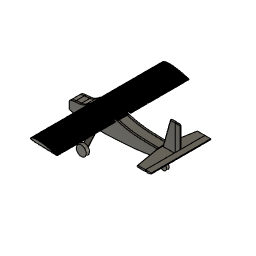
Arduino RC Plane - 3D Model (Autodesk Fusion 360 design; units mm, degrees)
Autodesk Fusion 360 part; units mm, degrees
(part 1 of 2)
sketch "Sketch1" plane through (0, 0, 0) normal (0, 1, 0) x (1, 0, 0)
  line L0 (95.8934, 1.764) -> (92.7195, 0.9111)
  line L1 (8.2584, 6.4801) -> (11.4851, 6.5775)
  line L2 (16.0241, -12.0922) -> (12.8008, -12.2387)
  line L3 (35.3144, -10.5067) -> (32.1062, -10.869)
  line L4 (14.7111, 6.6848) -> (17.9371, 6.7921)
  line L5 (12.8008, -12.2387) -> (9.5755, -12.3558)
  line L6 (37.2933, 7.4358) -> (40.5193, 7.5431)
  line L7 (34.0673, 7.3285) -> (37.2933, 7.4358)
  line L8 (27.6152, 7.114) -> (30.8412, 7.2213)
  line L9 (21.1632, 6.8994) -> (24.3892, 7.0067)
  line L10 (80.0088, -2.2846) -> (76.8274, -3.0295)
  line L11 (72.7795, 8.616) -> (76.0056, 8.7233)
  line L12 (40.5193, 7.5431) -> (43.7453, 7.6504)
  line L13 (38.5205, -10.1149) -> (35.3144, -10.5067)
  line L14 (88.9103, 9.1426) -> (92.1364, 9.2499)
  line L15 (24.3892, 7.0067) -> (27.6152, 7.114)
  line L16 (51.321, -8.2044) -> (48.1238, -8.7237)
  line L17 (-27.9436, -7.5856) -> (-29.6101, -6.8741)
  line L18 (44.9246, -9.2136) -> (41.7239, -9.6838)
  line L19 (92.1364, 9.2499) -> (95.3624, 9.3572)
  line L20 (53.4234, 7.9723) -> (56.6494, 8.0795)
  line L21 (-6.6136, -12.0485) -> (-9.8712, -11.7045)
  line L22 (-22.9804, -9.2004) -> (-26.284, -8.1991)
  line L23 (60.9003, -6.4698) -> (57.7093, -7.0774)
  line L24 (-11.0841, 5.6401) -> (-7.8642, 5.8357)
  line L25 (-30.3263, 3.3679) -> (-28.7346, 3.7257)
  line L26 (111.4925, 9.8936) -> (114.7185, 10.0009)
  line L27 (-23.9353, 4.4556) -> (-20.7278, 4.8278)
  line L28 (-3.3643, -12.2748) -> (-6.6136, -12.0485)
  line L29 (-33.4961, 2.4562) -> (-31.914, 2.9513)
  line L30 (59.8754, 8.1868) -> (63.1015, 8.2941)
  line L31 (56.6494, 8.0795) -> (59.8754, 8.1868)
  line L32 (-35.9566, 0.7068) -> (-35.3615, 1.3596)
  line L33 (118.0804, 8.1657) -> (114.9147, 7.1951)
  line L34 (-9.8712, -11.7045) -> (-13.1356, -11.2624)
  line L35 (9.5755, -12.3558) -> (6.3474, -12.4336)
  line L36 (30.8412, 7.2213) -> (34.0673, 7.3285)
  line L37 (108.5786, 5.3226) -> (105.4096, 4.4011)
  line L38 (48.1238, -8.7237) -> (44.9246, -9.2136)
  line L39 (50.1974, 7.865) -> (53.4234, 7.9723)
  line L40 (79.2323, 8.8207) -> (82.4583, 8.928)
  line L41 (63.1015, 8.2941) -> (66.3275, 8.4014)
  line L42 (22.4652, -11.7206) -> (19.246, -11.926)
  line L43 (122.7836, 10.2691) -> (125.1135, 10.3466)
  line L44 (-35.7385, -2.4129) -> (-36.0972, -1.9352)
  line L45 (-36.4605, -0.265) -> (-36.3957, -0.0633)
  line L46 (-17.5162, 5.1411) -> (-14.3018, 5.4151)
  line L47 (-35.0466, -3.1433) -> (-35.7385, -2.4129)
  line L48 (85.6843, 9.0353) -> (88.9103, 9.1426)
  line L49 (69.5535, 8.5087) -> (72.7795, 8.616)
  line L50 (5.0323, 6.3728) -> (8.2584, 6.4801)
  line L51 (122.8282, 9.6314) -> (121.2454, 9.1461)
  line L52 (28.8953, -11.1921) -> (25.6816, -11.476)
  line L53 (-36.0972, -1.9352) -> (-36.2873, -1.6133)
  line L54 (-7.8642, 5.8357) -> (-4.6423, 6.0019)
  line L55 (6.3474, -12.4336) -> (3.1152, -12.4526)
  line L56 (-27.138, 4.0148) -> (-23.9353, 4.4556)
  line L57 (98.5884, 9.4645) -> (101.8144, 9.5717)
  line L58 (57.7093, -7.0774) -> (54.5162, -7.6556)
  line L59 (125.1135, 10.3466) -> (122.8282, 9.6314)
  line L60 (-29.6101, -6.8741) -> (-31.2876, -6.0056)
  line L61 (119.5576, 10.1618) -> (121.1706, 10.2155)
  line L62 (64.0893, -5.8328) -> (60.9003, -6.4698)
  line L63 (92.7195, 0.9111) -> (89.5435, 0.0876)
  line L64 (-13.1356, -11.2624) -> (-16.4076, -10.7124)
  line L65 (111.747, 6.254) -> (108.5786, 5.3226)
  line L66 (119.6632, 8.651) -> (118.0804, 8.1657)
  line L67 (89.5435, 0.0876) -> (86.3669, -0.726)
  line L68 (121.1706, 10.2155) -> (122.7836, 10.2691)
  line L69 (-36.3957, -0.0633) -> (-36.2502, 0.2525)
  line L70 (-34.7442, 1.8366) -> (-33.4961, 2.4562)
  line L71 (76.0056, 8.7233) -> (79.2323, 8.8207)
  line L72 (114.9147, 7.1951) -> (111.747, 6.254)
  line L73 (-36.2873, -1.6133) -> (-36.3816, -1.3932)
  line L74 (95.3624, 9.3572) -> (98.5884, 9.4645)
  line L75 (67.2762, -5.1663) -> (64.0893, -5.8328)
  line L76 (102.2384, 3.5089) -> (99.0666, 2.6266)
  line L77 (-35.3615, 1.3596) -> (-34.7442, 1.8366)
  line L78 (-20.7278, 4.8278) -> (-17.5162, 5.1411)
  line L79 (114.7185, 10.0009) -> (117.9446, 10.1082)
  line L80 (-14.3018, 5.4151) -> (-11.0841, 5.6401)
  line L81 (-36.4861, -1.0259) -> (-36.4605, -0.265)
  line L82 (-31.2876, -6.0056) -> (-32.983, -4.882)
  line L83 (-34.3525, -3.7651) -> (-35.0466, -3.1433)
  line L84 (117.9446, 10.1082) -> (119.5576, 10.1618)
  line L85 (-32.983, -4.882) -> (-34.3525, -3.7651)
  line L86 (105.0405, 9.679) -> (108.2665, 9.7863)
  line L87 (-26.284, -8.1991) -> (-27.9436, -7.5856)
  line L88 (70.4618, -4.4802) -> (67.2762, -5.1663)
  line L89 (66.3275, 8.4014) -> (69.5535, 8.5087)
  line L90 (-28.7346, 3.7257) -> (-27.138, 4.0148)
  line L91 (-16.4076, -10.7124) -> (-19.6885, -10.0349)
  line L92 (108.2665, 9.7863) -> (111.4925, 9.8936)
  line L93 (43.7453, 7.6504) -> (46.9713, 7.7577)
  line L94 (76.8274, -3.0295) -> (73.6453, -3.7647)
  line L95 (54.5162, -7.6556) -> (51.321, -8.2044)
  line L96 (-36.3816, -1.3932) -> (-36.4861, -1.0259)
  line L97 (101.8144, 9.5717) -> (105.0405, 9.679)
  line L98 (105.4096, 4.4011) -> (102.2384, 3.5089)
  line L99 (46.9713, 7.7577) -> (50.1974, 7.865)
  line L100 (73.6453, -3.7647) -> (70.4618, -4.4802)
  line L101 (-36.2502, 0.2525) -> (-35.9566, 0.7068)
  line L102 (-31.914, 2.9513) -> (-30.3263, 3.3679)
  line L103 (99.0666, 2.6266) -> (95.8934, 1.764)
  line L104 (-1.4183, 6.1386) -> (1.8063, 6.2655)
  line L105 (83.1882, -1.5102) -> (80.0088, -2.2846)
  line L106 (86.3669, -0.726) -> (83.1882, -1.5102)
  line L107 (19.246, -11.926) -> (16.0241, -12.0922)
  line L108 (121.2454, 9.1461) -> (119.6632, 8.651)
  line L109 (-4.6423, 6.0019) -> (-1.4183, 6.1386)
  line L110 (25.6816, -11.476) -> (22.4652, -11.7206)
  line L111 (1.8063, 6.2655) -> (5.0323, 6.3728)
  line L112 (17.9371, 6.7921) -> (21.1632, 6.8994)
  line L113 (-19.6885, -10.0349) -> (-22.9804, -9.2004)
  line L114 (41.7239, -9.6838) -> (38.5205, -10.1149)
  line L115 (11.4851, 6.5775) -> (14.7111, 6.6848)
  line L116 (3.1152, -12.4526) -> (-0.1211, -12.4128)
  line L117 (82.4583, 8.928) -> (85.6843, 9.0353)
  line L118 (-0.1211, -12.4128) -> (-3.3643, -12.2748)
  line L119 (32.1062, -10.869) -> (28.8953, -11.1921)
  line L120 (433.5139, 105.8779) -> (-166.4861, 105.8779) construction
  line L121 (369.1135, 36.3466) -> (475.1135, 36.3466)
  line L122 (475.1135, 36.3466) -> (475.1135, 46.3466)
  line L123 (475.1135, 46.3466) -> (369.1135, 46.3466)
  line L124 (365.1135, 42.3466) -> (365.1135, 40.3466)
  arc A0 (365.1135, 40.3466) -> (369.1135, 36.3466) centre (369.1135, 40.3466) ccw
  arc A1 (369.1135, 46.3466) -> (365.1135, 42.3466) centre (369.1135, 42.3466) ccw
  line L125 (433.5395, 58.3466) -> (433.5395, 46.3466)
  line L126 (-36.4605, -0.265) -> (-72.4401, 24.9282)
  line L127 (-36.4605, -0.265) -> (0.5767, -0.265) construction
  line L128 (-101.6254, 35.5508) -> (-134.5473, 38.4311)
  line L129 (-166.4605, 53.4227) -> (-166.4605, 88.4227)
  spline S0 degree 5 poles (-158.5986, 98.1914) (-149.6531, 100.1493) (-132.0524, 103.7409) (-106.5214, 108.1556) (-73.5167, 112.2028) (-30.3842, 114.7027) (18.5122, 115.149) (75.7604, 113.8377) (140.9642, 110.664) (211.8798, 105.2223) (285.3301, 96.9119) (343.4794, 87.4326) (385.5551, 78.4692) (412.7641, 71.6318) (426.1581, 67.9976) knots 0 0 0 0 0 0 0.1 0.2 0.3 0.4 0.5 0.6 0.7 0.8 0.9 1 1 1 1 1 1
  line L130 (-201.7693, -33.0131) -> (-201.7693, 169.9869) construction
  line L131 (-201.7693, 68.4869) -> (-175.4519, 68.4869) construction
  arc A2 (-72.4401, 24.9282) -> (-101.6254, 35.5508) centre (-106.8547, -24.2209) ccw
  arc A3 (-159.8637, 44.0196) -> (-134.5473, 38.4311) centre (-125.8317, 138.0506) ccw
  arc A4 (-166.4605, 53.4227) -> (-159.8637, 44.0196) centre (-156.4605, 53.4227) ccw
  arc A5 (-158.5986, 98.1914) -> (-166.4605, 88.4227) centre (-156.4605, 88.4227) ccw
  arc A6 (433.5395, 58.3466) -> (426.1581, 67.9976) centre (423.5395, 58.3466) ccw
  line L132 (108.2665, 9.7863) -> (108.2665, 5.2318)
  spline S1 degree 5 poles (125.1135, 10.3466) (129.5122, 11.7241) (138.3251, 14.3811) (151.5908, 18.0725) (169.3737, 22.3977) (191.7903, 26.7637) (214.4829, 30.0801) (237.5863, 32.3933) (261.3798, 33.9707) (286.0084, 35.049) (311.4928, 35.7657) (332.5461, 36.1182) (348.6931, 36.2739) (359.614, 36.3302) (365.1135, 36.3466) knots 0 0 0 0 0 0 0.1 0.2 0.3 0.4 0.5 0.6 0.7 0.8 0.9 1 1 1 1 1 1
  line L133 (209.1359, 29.5835) -> (254.6924, 33.8044)
  line L134 (365.1135, 36.3466) -> (365.1135, 46.3466)
  spline S2 degree 5 poles (365.1135, 46.3466) (365.2736, 46.3477) (365.5937, 46.3495) (366.0739, 46.3513) (366.7139, 46.3521) (367.5139, 46.3513) (368.1538, 46.3498) (368.6336, 46.3483) (368.9536, 46.3472) (369.1135, 46.3466) knots 0 0 0 0 0 0 0.2 0.4 0.6 0.8 1 1 1 1 1 1
  line L135 (364.7053, 46.3438) -> (365.5217, 46.3493)
  line L136 (369.1135, 36.3466) -> (413.4661, -123.6534)
  line L137 (413.4661, -123.6534) -> (475.1135, -123.6534)
  line L138 (475.1135, -123.6534) -> (475.1135, 36.3466)
  point P0 (365.1135, 36.3466)
  point P1 (365.1135, 46.3466)
  point P2 (-85.6096, 34.1496)
  point P3 (-146.7743, 39.5008)
  point P4 (-166.4605, 100.9441)
  point P5 (19.9322, 114.7113)
  point P6 (433.5395, 70.3466)
  point P7 (231.9141, 31.694)
  dimension "d2" = 600
  dimension "d3" = 130
  dimension "d4" = 110
  dimension "d5" = 10
  dimension "d6" = 240
  dimension "d7" = 4
  dimension "d8" = 26
  dimension "d9" = 145
  dimension "d10" = 60
  dimension "d11" = 150
  dimension "d15" = 130
  dimension "d18" = 203
  dimension "d20" = 60
  dimension "d21" = 100
  dimension "d22" = 10
  dimension "d23" = 10
  dimension "d24" = 600
  dimension "d25" = 10
  dimension "d26" = 35
  dimension "d60" = 12
  dimension "d61" = 160
  constraint horizontal L120
  constraint horizontal L121
  constraint vertical L122
  constraint horizontal L123
  constraint vertical L124
  constraint coincident P0 L124
  constraint coincident P0 L121
  constraint tangent L124 A0
  constraint tangent L121 A0
  constraint coincident P1 L123
  constraint coincident P1 L124
  constraint tangent L123 A1
  constraint tangent L124 A1
  constraint equal A0 A1
  constraint coincident L123 L125.end
  constraint perpendicular L123 L125
  constraint horizontal L127
  constraint vertical L129
  constraint vertical L130
  constraint midpoint L130 L131.start
  constraint perpendicular L130 L131
  constraint coincident P2 L128
  constraint coincident P2 L126
  constraint tangent L128 A2
  constraint tangent L126 A2
  constraint coincident P3 L128
  constraint tangent L128 A3
  constraint tangent L129 A4
  constraint tangent A3 A4
  constraint coincident P4 L129
  constraint tangent L129 A5
  constraint tangent S0 A5
  constraint coincident L125 P6
  constraint tangent S0 A6
  constraint tangent L125 A6
  constraint vertical L132
  constraint coincident L37 L132.end
  constraint coincident P0 S1.end
  constraint midpoint P7 L133
  constraint coincident P1 L134.end
  constraint coincident L134 P1
  constraint midpoint P1 L135
  constraint perpendicular L125 L137
  constraint perpendicular L121 L138
  measures "d2" distance of L120.start L120.end
  measures "d3" horizontal distance of L81.start L120.end
  measures "d4" distance of P0 L121.end
  measures "d5" distance of P0 P1
  measures "d6" distance of L43.end L124
  measures "d7" radius of A0
  measures "d8" distance of L43.end L121
  measures "d9" angle of L126 L127
  measures "d10" distance of L45.start P2
  measures "d11" angle of L126 L128
  measures "d15" distance of L45.start L129
  measures "d18" distance of L130.start L130.end
  measures "d20" radius of A2
  measures "d21" radius of A3
  measures "d22" radius of A4
  measures "d23" radius of A5
  measures "d24" distance of L125 L129
  measures "d25" radius of A6
  measures "d26" distance of L129.start L129.end
  measures "d60" distance of L125.end L125.start
  measures "d61" distance of L121.end L137.end
extrude "Extrude1" add sketch "Sketch1" along normal mid plane 800 contours L0 L1 L2 L3 L4 L5 L6 L7 L8 L9 L10 L11 L12 L13 L14 L15 L16 L17 L18 L19 L20 L21 L22 L23 L24 L25 L27 L28 L29 L30 L31 L32 L34 L35 L36 L37 L38 L39 L40 L41 L42 L44 L45 L46 L47 L48 L49 L50 L52 L53 L54 L55 L56 L57 L58 L60 L62 L63 L64 L67 L69 L70 L71 L73 L74 L75 L76 L77 L78 L80 L81 L82 L83 L85 L86 L87 L88 L89 L90 L91 L93 L94 L95 L96 L97 L98 L99 L100 L101 L102 L103 L104 L105 L106 L107 L109 L110 L111 L112 L113 L114 L115 L116 L117 L118 L119 L132 | L26 L33 L37 L43 L51 L59 L61 L65 L66 L68 L72 L79 L84 L92 L108 L132 makes body 1
copy_body "Body->Comp2" bodies 1 removing the originals makes body 2 in component "Component"
extrude "Extrude1'" add sketch "Sketch1" along normal blind 45 separate body contours L1 L4 L6 L7 L8 L9 L11 L12 L14 L15 L19 L20 L24 L25 L26 L27 L29 L30 L31 L32 L36 L39 L40 L41 L43 L45 L46 L48 L49 L50 L54 L56 L57 L61 L68 L69 L70 L71 L74 L77 L78 L79 L80 L84 L86 L89 L90 L92 L93 L97 L99 L101 L102 L104 L109 L111 L112 L115 L117 L123 L124 L125 L126 L128 L129 S0 A2 A3 A4 A5 A6 S1 L134 S2 L135 makes body 3 in component "Component'"
extrude "Extrude2" cut sketch "Sketch1" along normal blind 25 contours L1 L4 L6 L7 L8 L9 L11 L12 L14 L15 L19 L20 L24 L25 L26 L27 L29 L30 L31 L32 L36 L39 L40 L41 L43 L45 L46 L48 L49 L50 L54 L56 L57 L61 L68 L69 L70 L71 L74 L77 L78 L79 L80 L84 L86 L89 L90 L92 L93 L97 L99 L101 L102 L104 L109 L111 L112 L115 L117 L123 L124 L125 L126 L128 L129 S0 A2 A3 A4 A5 A6 S1 L134 S2 L135 bodies 3 in component "Component'"
sketch "Sketch1 (2)" plane through (0, 0, 0) normal (0, 1, 0) x (1, 0, 0) in component "Component''"
  line L0 (433.5395, 58.3466) -> (433.5395, 46.3466)
  line L1 (433.5395, 46.3466) -> (369.1135, 46.3466)
  spline S0 degree 3 poles (365.1135, 46.3466) (365.7936, 46.3512) (366.4616, 46.3521) (367.7595, 46.351) (368.4873, 46.3489) (369.1135, 46.3466) knots -0.377645 -0.377645 -0.377645 -0.377645 -0.187855 -0.187855 0 0 0 0
  line L2 (125.1135, 10.3466) -> (122.7836, 10.2691)
  line L3 (122.7836, 10.2691) -> (114.7185, 10.0009)
  line L4 (114.7185, 10.0009) -> (111.4925, 9.8936)
  line L5 (111.4925, 9.8936) -> (105.0405, 9.679)
  line L6 (105.0405, 9.679) -> (101.8144, 9.5717)
  line L7 (101.8144, 9.5717) -> (98.5884, 9.4645)
  line L8 (98.5884, 9.4645) -> (79.2323, 8.8207)
  line L9 (79.2323, 8.8207) -> (76.0056, 8.7233)
  line L10 (76.0056, 8.7233) -> (72.7795, 8.616)
  line L11 (72.7795, 8.616) -> (69.5535, 8.5087)
  line L12 (69.5535, 8.5087) -> (66.3275, 8.4014)
  line L13 (66.3275, 8.4014) -> (63.1015, 8.2941)
  line L14 (63.1015, 8.2941) -> (59.8754, 8.1868)
  line L15 (59.8754, 8.1868) -> (56.6494, 8.0795)
  line L16 (56.6494, 8.0795) -> (53.4234, 7.9723)
  line L17 (53.4234, 7.9723) -> (50.1974, 7.865)
  line L18 (50.1974, 7.865) -> (46.9713, 7.7577)
  line L19 (46.9713, 7.7577) -> (43.7453, 7.6504)
  line L20 (43.7453, 7.6504) -> (40.5193, 7.5431)
  line L21 (40.5193, 7.5431) -> (37.2933, 7.4358)
  line L22 (37.2933, 7.4358) -> (34.0673, 7.3285)
  line L23 (34.0673, 7.3285) -> (30.8412, 7.2213)
  line L24 (30.8412, 7.2213) -> (27.6152, 7.114)
  line L25 (27.6152, 7.114) -> (24.3892, 7.0067)
  line L26 (24.3892, 7.0067) -> (21.1632, 6.8994)
  line L27 (21.1632, 6.8994) -> (17.9371, 6.7921)
  line L28 (17.9371, 6.7921) -> (11.4851, 6.5775)
  line L29 (11.4851, 6.5775) -> (8.2584, 6.4801)
  line L30 (8.2584, 6.4801) -> (1.8063, 6.2655)
  line L31 (1.8063, 6.2655) -> (-1.4183, 6.1386)
  line L32 (-1.4183, 6.1386) -> (-4.6423, 6.0019)
  line L33 (-4.6423, 6.0019) -> (-7.8642, 5.8357)
  line L34 (-7.8642, 5.8357) -> (-11.0841, 5.6401)
  line L35 (-11.0841, 5.6401) -> (-14.3018, 5.4151)
  line L36 (-14.3018, 5.4151) -> (-17.5162, 5.1411)
  line L37 (-17.5162, 5.1411) -> (-20.7278, 4.8278)
  line L38 (-20.7278, 4.8278) -> (-23.9353, 4.4556)
  line L39 (-23.9353, 4.4556) -> (-27.138, 4.0148)
  line L40 (-27.138, 4.0148) -> (-28.7346, 3.7257)
  line L41 (-28.7346, 3.7257) -> (-30.3263, 3.3679)
  line L42 (-30.3263, 3.3679) -> (-31.914, 2.9513)
  line L43 (-31.914, 2.9513) -> (-33.4961, 2.4562)
  line L44 (-33.4961, 2.4562) -> (-34.7442, 1.8366)
  line L45 (-34.7442, 1.8366) -> (-35.3615, 1.3596)
  line L46 (-35.3615, 1.3596) -> (-35.9566, 0.7068)
  line L47 (-35.9566, 0.7068) -> (-36.2502, 0.2525)
  line L48 (-36.2502, 0.2525) -> (-36.3957, -0.0633)
  line L49 (-36.3957, -0.0633) -> (-36.4605, -0.265)
  line L50 (-36.4605, -0.265) -> (-72.4401, 24.9282)
  arc A0 (-72.4401, 24.9282) -> (-101.6254, 35.5508) centre (-106.8547, -24.2209) ccw
  line L51 (-101.6254, 35.5508) -> (-134.5473, 38.4311)
  arc A1 (-159.8637, 44.0196) -> (-134.5473, 38.4311) centre (-125.8317, 138.0506) ccw
  arc A2 (-166.4605, 53.4227) -> (-159.8637, 44.0196) centre (-156.4605, 53.4227) ccw
  line L52 (-166.4605, 53.4227) -> (-166.4605, 88.4227)
  arc A3 (-158.5986, 98.1914) -> (-166.4605, 88.4227) centre (-156.4605, 88.4227) ccw
  spline S1 degree 3 poles (426.1581, 67.9976) (374.7187, 81.9546) (317.2109, 92.6975) (193.3206, 107.1118) (132.9422, 111.3091) (17.9002, 115.6029) (-23.1255, 114.8448) (-84.5053, 111.2062) (-117.7698, 107.1276) (-158.5986, 98.1914) knots -44.857348 -44.857348 -44.857348 -44.857348 -33.005579 -33.005579 -23.298988 -23.298988 -12.538582 -12.538582 0 0 0 0
  arc A4 (433.5395, 58.3466) -> (426.1581, 67.9976) centre (423.5395, 58.3466) ccw
  line L53 (-23.9353, 4.4556) -> (-23.9353, 16.5361)
  line L54 (-154.4605, 54.8376) -> (-154.4605, 86.8115)
  line L55 (123.2114, 22.29) -> (122.3848, 22.2625)
  line L56 (122.3848, 22.2625) -> (114.3197, 21.9943)
  line L57 (114.3197, 21.9943) -> (111.0937, 21.887)
  line L58 (111.0937, 21.887) -> (104.6416, 21.6724)
  line L59 (104.6416, 21.6724) -> (101.4156, 21.5651)
  line L60 (101.4156, 21.5651) -> (98.1896, 21.4578)
  line L61 (98.1896, 21.4578) -> (78.8517, 20.8147)
  line L62 (78.8517, 20.8147) -> (75.625, 20.7172)
  line L63 (75.625, 20.7172) -> (72.3807, 20.6093)
  line L64 (72.3807, 20.6093) -> (69.1547, 20.5021)
  line L65 (69.1547, 20.5021) -> (65.9286, 20.3948)
  line L66 (65.9286, 20.3948) -> (62.7026, 20.2875)
  line L67 (62.7026, 20.2875) -> (59.4766, 20.1802)
  line L68 (59.4766, 20.1802) -> (56.2506, 20.0729)
  line L69 (56.2506, 20.0729) -> (53.0245, 19.9656)
  line L70 (53.0245, 19.9656) -> (49.7985, 19.8583)
  line L71 (49.7985, 19.8583) -> (46.5725, 19.7511)
  line L72 (46.5725, 19.7511) -> (43.3465, 19.6438)
  line L73 (43.3465, 19.6438) -> (40.1204, 19.5365)
  line L74 (40.1204, 19.5365) -> (36.8944, 19.4292)
  line L75 (36.8944, 19.4292) -> (33.6684, 19.3219)
  line L76 (33.6684, 19.3219) -> (30.4424, 19.2146)
  line L77 (30.4424, 19.2146) -> (27.2163, 19.1073)
  line L78 (27.2163, 19.1073) -> (23.9903, 19.0001)
  line L79 (23.9903, 19.0001) -> (20.7643, 18.8928)
  line L80 (20.7643, 18.8928) -> (17.5383, 18.7855)
  line L81 (17.5383, 18.7855) -> (11.1045, 18.5715)
  line L82 (11.1045, 18.5715) -> (7.8778, 18.474)
  line L83 (7.8778, 18.474) -> (1.3709, 18.2577)
  line L84 (1.3709, 18.2577) -> (-1.9085, 18.1286)
  line L85 (-1.9085, 18.1286) -> (-5.2055, 17.9888)
  line L86 (-5.2055, 17.9888) -> (-8.537, 17.817)
  line L87 (-8.537, 17.817) -> (-11.8664, 17.6147)
  line L88 (-11.8664, 17.6147) -> (-15.2302, 17.3795)
  line L89 (-15.2302, 17.3795) -> (-18.6085, 17.0915)
  line L90 (-18.6085, 17.0915) -> (-22.002, 16.7604)
  line L91 (-22.002, 16.7604) -> (-25.4452, 16.3609)
  line L92 (-25.4452, 16.3609) -> (-29.0261, 15.868)
  line L93 (-29.0261, 15.868) -> (-31.1204, 15.4888)
  line L94 (-31.1204, 15.4888) -> (-33.1659, 15.0291)
  line L95 (-33.1659, 15.0291) -> (-35.2306, 14.4872)
  line L96 (-35.2306, 14.4872) -> (-36.1822, 14.1895)
  line L97 (-36.1822, 14.1895) -> (-65.5572, 34.7581)
  arc A5 (-65.5572, 34.7581) -> (-100.5795, 47.5051) centre (-106.8547, -24.2209) ccw
  line L98 (-100.5795, 47.5051) -> (-133.5015, 50.3854)
  arc A6 (-154.4605, 54.8376) -> (-133.5015, 50.3854) centre (-125.8317, 138.0506) ccw
  line L99 (101.8144, 9.5717) -> (101.8144, 21.5784)
  line L100 (-150.921, 57.3732) -> (-120.921, 57.3732)
  line L101 (-120.921, 57.3732) -> (-120.921, 85.3732)
  line L102 (-120.921, 85.3732) -> (-150.921, 85.3732)
  line L103 (-150.921, 85.3732) -> (-150.921, 57.3732)
  line L104 (78.6971, 49.721) -> (100.6971, 49.721)
  line L105 (100.6971, 49.721) -> (100.6971, 75.721)
  line L106 (100.6971, 75.721) -> (78.6971, 75.721)
  line L107 (78.6971, 75.721) -> (78.6971, 49.721)
  line L108 (153.5395, 91.8115) -> (153.5395, 30.6156)
  line L109 (-166.4605, 53.4227) -> (-166.4605, 88.4227)
  line L110 (173.5395, -153.5975) -> (173.5395, 198.2659) construction
  line L111 (-154.4605, 86.8115) -> (-131.4605, 86.8115)
  spline S2 degree 3 poles (123.2114, 22.29) (133.5497, 25.285) (143.6571, 28.0575) (153.5395, 30.6156) knots -26.624685 -26.624685 -26.624685 -26.624685 -23.3972 -23.3972 -23.3972 -23.3972
  line L112 (365.1135, 46.3466) -> (365.1135, 36.3466)
  spline S3 degree 3 poles (125.1135, 10.3466) (172.1032, 25.0618) (209.4342, 29.8358) (274.1497, 35.2585) (322.4324, 36.2198) (365.1135, 36.3466) knots -22.769958 -22.769958 -22.769958 -22.769958 -12.804404 -12.804404 0 0 0 0
  line L113 (-131.4605, 86.8115) -> (-131.4605, 91.8115)
  line L114 (-131.4605, 91.8115) -> (153.5395, 91.8115)
  dimension "d44" = 30
  dimension "d45" = 28
  dimension "d46" = 22
  dimension "d47" = 26
  dimension "d48" = 320
  dimension "d49" = 340
  dimension "d146" = 5
  dimension "d147" = 35
  constraint coincident L38.end L39.start
  constraint vertical L53
  constraint coincident L53.end L91
  constraint vertical L99
  constraint coincident L6.end L7.start
  constraint coincident L59 L99.end
  constraint horizontal L100
  constraint vertical L101
  constraint horizontal L102
  constraint vertical L103
  constraint horizontal L111
  constraint horizontal L104
  constraint vertical L105
  constraint horizontal L106
  constraint vertical L107
  constraint vertical L108
  constraint vertical L110
  constraint parallel L52 L54
  constraint parallel L2 L55
  constraint parallel L3 L56
  constraint parallel L4 L57
  constraint parallel L5 L58
  constraint parallel L6 L59
  constraint parallel L7 L60
  constraint parallel L8 L61
  constraint parallel L9 L62
  constraint parallel L10 L63
  constraint parallel L11 L64
  constraint parallel L12 L65
  constraint parallel L13 L66
  constraint parallel L14 L67
  constraint parallel L15 L68
  constraint parallel L16 L69
  constraint parallel L17 L70
  constraint parallel L18 L71
  constraint parallel L19 L72
  constraint parallel L20 L73
  constraint parallel L21 L74
  constraint parallel L22 L75
  constraint parallel L23 L76
  constraint parallel L24 L77
  constraint parallel L25 L78
  constraint parallel L26 L79
  constraint parallel L27 L80
  constraint parallel L28 L81
  constraint parallel L29 L82
  constraint parallel L30 L83
  constraint parallel L31 L84
  constraint parallel L32 L85
  constraint parallel L33 L86
  constraint parallel L34 L87
  constraint parallel L35 L88
  constraint parallel L36 L89
  constraint parallel L37 L90
  constraint parallel L38 L91
  constraint parallel L39 L92
  constraint parallel L40 L93
  constraint parallel L41 L94
  constraint parallel L42 L95
  constraint parallel L43 L96
  constraint parallel L50 L97
  constraint concentric A0 A5
  constraint parallel L51 L98
  constraint concentric A1 A6
  constraint tangent A5 L98
  constraint tangent L97 A5
  constraint tangent L98 A6
  constraint vertical L113
  constraint perpendicular L108 L114
  measures "d44" distance of L100.start L100.end
  measures "d45" distance of L100.start L102.end
  measures "d46" distance of L104.start L104.end
  measures "d47" distance of L104.start L106.end
  measures "d48" distance of L108 L109
  measures "d49" distance of L109 L110
  measures "d146" distance of L111.end L113.end
  measures "d147" distance of L109 L113
ref_plane "WorkPlane1" through (0, 25, 0) normal (0, 1, 0) x (-1, 0, 0)
extrude "Extrude1''" add sketch "Sketch1 (2)" along normal mid plane 50 separate body contours L0 L1 S0 L2 L3 L4 L5 L6 L39 L40 L41 L42 L43 L44 L45 L46 L47 L48 L49 L50 A0 L51 A1 A2 L52 A3 S1 A4 L53 L54 L55 L56 L57 L58 L59 L91 L92 L93 L94 L95 L96 L97 A5 L98 A6 L99 L108 L109 L111 S2 L112 S3 L113 L114 makes body 4 in component "Component''"
extrude "Extrude1'''" add sketch "Sketch1" along normal mid plane 360 separate body contours L121 L122 L123 L124 A0 A1 L134 makes body 5 in component "Component'''"
extrude "Extrude3" add sketch "Sketch1" along normal blind 45 contours L26 L33 L37 L43 L51 L59 L61 L65 L66 L68 L72 L79 L84 L92 L108 L132 bodies 3 in component "Component'"
extrude "Extrude4" cut sketch "Sketch1" along normal blind 25 contours L26 L33 L37 L43 L51 L59 L61 L65 L66 L68 L72 L79 L84 L92 L108 L132 bodies 3 in component "Component'"
extrude "Extrude2'" add sketch "Sketch1" along normal mid plane 50 contours L26 L33 L37 L43 L51 L59 L61 L65 L66 L68 L72 L79 L84 L92 L108 L132 bodies 4 in component "Component''"
extrude "Extrude1''''" add sketch "Sketch1" along normal mid plane 10 separate body contours L121 L136 L137 L138 makes body 6 in component "Component''''"
sketch "Sketch2" plane through (0, 0, -36.3466) normal (0, 0, 1) x (-1, 0, 0)
  line L0 (-475.1135, 180) -> (-475.1135, -180)
  line L1 (-475.1135, -180) -> (-369.1135, -180)
  line L2 (-369.1135, -180) -> (-369.1135, 180)
  line L3 (-369.1135, 180) -> (-475.1135, 180)
  line L4 (-369.1135, 180) -> (-369.1135, -180)
  line L5 (-369.1135, -180) -> (-365.1135, -180)
  line L6 (-365.1135, -180) -> (-365.1135, 180)
  line L7 (-365.1135, 180) -> (-369.1135, 180)
  line L8 (-365.1135, 180) -> (-365.1135, -180)
  line L9 (-365.1135, 180) -> (-390.1135, 180)
  line L10 (-365.1135, 40) -> (-390.1135, 180)
  line L11 (-365.1135, -40) -> (-390.1135, -180)
  line L12 (-365.1135, -180) -> (-390.1135, -180)
  dimension "d67" = 25
  dimension "d68" = 140
  dimension "d69" = 25
  dimension "d70" = 140
  constraint coincident L6.end L7.start
  constraint coincident L3 L9.end
  constraint perpendicular L6 L9
  constraint coincident L6 L10.start
  constraint coincident L8 L11.start
  constraint coincident L1 L11.end
  constraint coincident L5.end L6.start
  measures "d67" distance of L6.end L9.end
  measures "d68" distance of L9 L10.start
  measures "d69" distance of L11.end L5.end
  measures "d70" distance of L11.start L5.end
extrude "Extrude2''" cut sketch "Sketch2" against normal blind 13 contours L2 L3 L4 L9 L10 | L1 L2 L4 L11 L12 | L2 L4 L6 L7 L8 L9 L10 | L2 L4 L5 L6 L8 L11 L12 bodies 5 in component "Component'''"
fillet "Fillet2" radius 4 10 edges at (379.6135, -121.2, -46.3466) (366.2851, -46.5608, -45.175) (365.1135, -40, -41.3466) (366.2851, -46.5608, -37.5182) (379.6135, -121.2, -36.3466) (379.6135, 121.2, -36.3466) (366.2851, 46.5608, -37.5182) (365.1135, 40, -41.3466) (366.2851, 46.5608, -45.175) (379.6135, 121.2, -46.3466) on bodies 5 in component "Component'''"
fillet "Fillet1" radius 4 2 edges at (391.2898, -5, 43.6534) (391.2898, 5, 43.6534) on bodies 6 in component "Component''''"
sketch "Sketch3" plane through (0, -180, 0) normal (0, -1, 0) x (1, 0, 0)
  ellipse E0 centre (394.1768, -42.3466) end of major axis (390.1135, -42.3466) minor radius 4 (390.1135, -42.3466) -> (394.1768, -46.3466) ccw
  line L0 (394.1768, -46.3466) -> (475.1135, -46.3466)
  line L1 (475.1135, -46.3466) -> (475.1135, -36.3466)
  line L2 (475.1135, -36.3466) -> (394.1768, -36.3466)
  ellipse E1 centre (394.1768, -40.3466) end of major axis (390.1135, -40.3466) minor radius 4 (394.1768, -36.3466) -> (390.1135, -40.3466) ccw
  line L3 (390.1135, -40.3466) -> (390.1135, -42.3466)
  line L4 (440.1135, -36.3466) -> (440.1135, -46.3466)
  line L5 (440.1135, -36.3466) -> (450.1135, -46.3466)
  line L6 (440.1135, -36.3466) -> (440.7895, -36.3466) construction
  line L7 (440.1135, -46.3466) -> (450.1135, -46.3466)
  line L8 (475.1135, -41.3466) -> (460.1135, -46.3466)
  line L9 (460.1135, -46.3466) -> (475.1135, -46.3466)
  line L10 (475.1135, -46.3466) -> (475.1135, -41.3466)
  dimension "d73" = 45
  dimension "d74" = 35
  dimension "d77" = 5
  dimension "d78" = 15
  constraint coincident L2 L4.start
  constraint coincident L0 L4.end
  constraint perpendicular L0 L4
  constraint horizontal L6
  constraint coincident L0 L5.end
  constraint coincident L1 L8.start
  constraint coincident L0 L8.end
  constraint coincident L0.end L1.start
  measures "d73" angle of L5 L6
  measures "d74" distance of L1 L4
  measures "d77" distance of L0 L8.start
  measures "d78" distance of L0.end L8.end
extrude "Extrude3'" cut sketch "Sketch3" against normal blind 360 contours L0 L4 L5 L7 | L0 L1 L8 L9 L10 bodies 5 in component "Component'''"
sketch "Sketch4" plane through (0, -5, 0) normal (0, -1, 0) x (1, 0, 0)
  line L0 (417.6169, 123.6534) -> (373.2643, -36.3466)
  line L1 (373.2643, -36.3466) -> (475.1135, -36.3466)
  line L2 (475.1135, -36.3466) -> (475.1135, 123.6534)
  line L3 (475.1135, 123.6534) -> (417.6169, 123.6534)
  line L4 (440.1135, -36.3466) -> (475.1135, -1.3466)
  line L5 (440.1135, -36.3466) -> (475.1135, -36.3466)
  line L6 (475.1135, -1.3466) -> (475.1135, -36.3466)
  dimension "d79" = 35
  dimension "d80" = 45
  constraint coincident L1 L4.start
  constraint coincident L2 L4.end
  constraint coincident L1.end L2.start
  measures "d79" distance of L4.start L1.end
  measures "d80" angle of L4 L5
extrude "Extrude2'''" cut sketch "Sketch4" against normal blind 10 contours L1 L2 L4 L5 L6 bodies 6 in component "Component''''"
sketch "Sketch5" plane through (0, 0, 123.6534) normal (0, 0, 1) x (-1, 0, 0)
  ellipse E0 centre (-417.6169, -1) end of major axis (-413.4661, -1) minor radius 4 (-417.6169, -5) -> (-413.4661, -1) ccw
  line L0 (-413.4661, -1) -> (-413.4661, 1)
  ellipse E1 centre (-417.6169, 1) end of major axis (-413.4661, 1) minor radius 4 (-413.4661, 1) -> (-417.6169, 5) ccw
  line L1 (-417.6169, 5) -> (-475.1135, 5)
  line L2 (-475.1135, 5) -> (-475.1135, -5)
  line L3 (-475.1135, -5) -> (-417.6169, -5)
  line L4 (-445.1135, -5) -> (-445.1135, 5)
  line L5 (-460.1135, -5) -> (-475.1135, 0)
  line L6 (-445.1135, 5) -> (-455.1135, -5)
  dimension "d83" = 30
  dimension "d85" = 45
  dimension "d86" = 15
  dimension "d87" = 5
  constraint coincident L3 L4.start
  constraint coincident L1 L4.end
  constraint perpendicular L1 L4
  constraint coincident L3 L5.start
  constraint coincident L2 L5.end
  constraint coincident L3 L6.end
  measures "d83" distance of L2 L4
  measures "d85" angle of L4 L6
  measures "d86" distance of L2 L5.start
  measures "d87" distance of L3 L5.end
extrude "Extrude3''" cut sketch "Sketch5" against normal up to surface (160 mm away) contours L3 L4 L6 | L2 L3 L5 bodies 6 in component "Component''''"
sketch "Sketch7" plane through (0, 0, 0) normal (0, 1, 0) x (1, 0, 0)
  line L0 (108.2665, 9.7863) -> (108.2665, 5.2318)
  line L1 (105.0405, 9.679) -> (111.4925, 9.8936)
  line L2 (111.4925, 9.8936) -> (114.7185, 10.0009)
  line L3 (114.7185, 10.0009) -> (122.7836, 10.2691)
  line L4 (122.7836, 10.2691) -> (125.1135, 10.3466)
  line L5 (125.1135, 10.3466) -> (122.8282, 9.6314)
  line L6 (122.8282, 9.6314) -> (121.2454, 9.1461)
  line L7 (121.2454, 9.1461) -> (119.6632, 8.651)
  line L8 (119.6632, 8.651) -> (118.0804, 8.1657)
  line L9 (118.0804, 8.1657) -> (114.9147, 7.1951)
  line L10 (114.9147, 7.1951) -> (111.747, 6.254)
  line L11 (111.747, 6.254) -> (108.5786, 5.3226)
  line L12 (108.5786, 5.3226) -> (105.4096, 4.4011)
extrude "Extrude1'''''" cut sketch "Sketch7" along normal mid plane 90 bodies 2 in component "Component"
ref_plane "WorkPlane2" through (133.5395, -145, -57.669) normal (0, -1, 0) x (-1, 0, 0)
sketch "Sketch8" plane through (133.5395, -145, -57.669) normal (0, -1, 0) x (1, 0, 0)
  line L0 (-48.426, 58.7102) -> (-48.426, 48.6526)
  line L1 (-98.2251, 68.1756) -> (-101.4333, 68.538)
  line L2 (-101.4333, 68.538) -> (-104.6442, 68.8611)
  line L3 (-104.6442, 68.8611) -> (-107.8579, 69.1449)
  line L4 (-107.8579, 69.1449) -> (-111.0743, 69.3896)
  line L5 (-111.0743, 69.3896) -> (-114.2935, 69.595)
  line L6 (-114.2935, 69.595) -> (-117.5154, 69.7611)
  line L7 (-117.5154, 69.7611) -> (-120.7387, 69.9076)
  line L8 (-120.7387, 69.9076) -> (-123.964, 70.0247)
  line L9 (-123.964, 70.0247) -> (-127.1921, 70.1026)
  line L10 (-127.1921, 70.1026) -> (-130.4243, 70.1216)
  line L11 (-130.4243, 70.1216) -> (-133.6606, 70.0817)
  line L12 (-133.6606, 70.0817) -> (-136.9038, 69.9437)
  line L13 (-136.9038, 69.9437) -> (-140.1531, 69.7175)
  line L14 (-140.1531, 69.7175) -> (-143.4107, 69.3735)
  line L15 (-143.4107, 69.3735) -> (-146.6752, 68.9314)
  line L16 (-146.6752, 68.9314) -> (-149.9472, 68.3814)
  line L17 (-149.9472, 68.3814) -> (-153.2281, 67.7038)
  line L18 (-153.2281, 67.7038) -> (-156.5199, 66.8693)
  line L19 (-156.5199, 66.8693) -> (-159.8235, 65.8681)
  line L20 (-159.8235, 65.8681) -> (-161.4831, 65.2546)
  line L21 (-161.4831, 65.2546) -> (-163.1497, 64.543)
  line L22 (-163.1497, 64.543) -> (-164.8272, 63.6745)
  line L23 (-164.8272, 63.6745) -> (-166.5225, 62.5509)
  line L24 (-166.5225, 62.5509) -> (-167.892, 61.4341)
  line L25 (-167.892, 61.4341) -> (-168.5862, 60.8123)
  line L26 (-168.5862, 60.8123) -> (-169.278, 60.0818)
  line L27 (-169.278, 60.0818) -> (-169.6367, 59.6042)
  line L28 (-169.6367, 59.6042) -> (-169.8268, 59.2823)
  line L29 (-169.8268, 59.2823) -> (-169.9211, 59.0621)
  line L30 (-169.9211, 59.0621) -> (-170.0257, 58.6948)
  line L31 (-170.0257, 58.6948) -> (-170, 57.9339)
  line L32 (-170, 57.9339) -> (-169.9352, 57.7322)
  line L33 (-169.9352, 57.7322) -> (-169.7897, 57.4165)
  line L34 (-169.7897, 57.4165) -> (-169.4962, 56.9622)
  line L35 (-169.4962, 56.9622) -> (-168.901, 56.3093)
  line L36 (-168.901, 56.3093) -> (-168.2837, 55.8324)
  line L37 (-168.2837, 55.8324) -> (-167.0356, 55.2128)
  line L38 (-167.0356, 55.2128) -> (-165.4535, 54.7177)
  line L39 (-165.4535, 54.7177) -> (-163.8659, 54.301)
  line L40 (-163.8659, 54.301) -> (-162.2741, 53.9433)
  line L41 (-162.2741, 53.9433) -> (-160.6776, 53.6542)
  line L42 (-160.6776, 53.6542) -> (-157.4749, 53.2133)
  line L43 (-157.4749, 53.2133) -> (-154.2674, 52.8412)
  line L44 (-154.2674, 52.8412) -> (-151.0557, 52.5279)
  line L45 (-151.0557, 52.5279) -> (-147.8414, 52.2538)
  line L46 (-147.8414, 52.2538) -> (-144.6236, 52.0288)
  line L47 (-144.6236, 52.0288) -> (-141.4037, 51.8332)
  line L48 (-141.4037, 51.8332) -> (-138.1818, 51.6671)
  line L49 (-138.1818, 51.6671) -> (-134.9579, 51.5304)
  line L50 (-134.9579, 51.5304) -> (-131.7332, 51.4035)
  line L51 (-131.7332, 51.4035) -> (-125.2812, 51.1889)
  line L52 (-125.2812, 51.1889) -> (-122.0544, 51.0914)
  line L53 (-122.0544, 51.0914) -> (-115.6024, 50.8768)
  line L54 (-115.6024, 50.8768) -> (-112.3764, 50.7695)
  line L55 (-112.3764, 50.7695) -> (-109.1503, 50.6623)
  line L56 (-109.1503, 50.6623) -> (-105.9243, 50.555)
  line L57 (-105.9243, 50.555) -> (-102.6983, 50.4477)
  line L58 (-102.6983, 50.4477) -> (-99.4723, 50.3404)
  line L59 (-99.4723, 50.3404) -> (-96.2462, 50.2331)
  line L60 (-96.2462, 50.2331) -> (-93.0202, 50.1258)
  line L61 (-93.0202, 50.1258) -> (-89.7942, 50.0185)
  line L62 (-89.7942, 50.0185) -> (-86.5682, 49.9113)
  line L63 (-86.5682, 49.9113) -> (-83.3422, 49.804)
  line L64 (-83.3422, 49.804) -> (-80.1161, 49.6967)
  line L65 (-80.1161, 49.6967) -> (-76.8901, 49.5894)
  line L66 (-76.8901, 49.5894) -> (-73.6641, 49.4821)
  line L67 (-73.6641, 49.4821) -> (-70.4381, 49.3748)
  line L68 (-70.4381, 49.3748) -> (-67.212, 49.2675)
  line L69 (-67.212, 49.2675) -> (-63.986, 49.1603)
  line L70 (-63.986, 49.1603) -> (-60.76, 49.053)
  line L71 (-60.76, 49.053) -> (-57.534, 48.9457)
  line L72 (-57.534, 48.9457) -> (-54.3072, 48.8482)
  line L73 (-54.3072, 48.8482) -> (-34.9511, 48.2045)
  line L74 (-34.9511, 48.2045) -> (-31.7251, 48.0972)
  line L75 (-31.7251, 48.0972) -> (-28.499, 47.9899)
  line L76 (-28.499, 47.9899) -> (-22.047, 47.7754)
  line L77 (-22.047, 47.7754) -> (-18.821, 47.6681)
  line L78 (-18.821, 47.6681) -> (-10.7559, 47.3999)
  line L79 (-10.7559, 47.3999) -> (-8.426, 47.3224)
  line L80 (-8.426, 47.3224) -> (-10.7113, 48.0375)
  line L81 (-10.7113, 48.0375) -> (-12.2942, 48.5228)
  line L82 (-12.2942, 48.5228) -> (-13.8763, 49.0179)
  line L83 (-13.8763, 49.0179) -> (-15.4591, 49.5032)
  line L84 (-15.4591, 49.5032) -> (-18.6248, 50.4738)
  line L85 (-18.6248, 50.4738) -> (-21.7925, 51.415)
  line L86 (-21.7925, 51.415) -> (-24.9609, 52.3463)
  line L87 (-24.9609, 52.3463) -> (-28.13, 53.2679)
  line L88 (-28.13, 53.2679) -> (-31.3011, 54.16)
  line L89 (-31.3011, 54.16) -> (-34.473, 55.0423)
  line L90 (-34.473, 55.0423) -> (-37.6462, 55.905)
  line L91 (-37.6462, 55.905) -> (-40.8201, 56.7579)
  line L92 (-40.8201, 56.7579) -> (-43.996, 57.5813)
  line L93 (-43.996, 57.5813) -> (-47.1726, 58.3949)
  line L94 (-47.1726, 58.3949) -> (-50.3513, 59.1791)
  line L95 (-50.3513, 59.1791) -> (-53.5307, 59.9535)
  line L96 (-53.5307, 59.9535) -> (-56.7121, 60.6985)
  line L97 (-56.7121, 60.6985) -> (-59.8942, 61.4336)
  line L98 (-59.8942, 61.4336) -> (-63.0777, 62.1492)
  line L99 (-63.0777, 62.1492) -> (-66.2633, 62.8353)
  line L100 (-66.2633, 62.8353) -> (-69.4502, 63.5017)
  line L101 (-69.4502, 63.5017) -> (-72.6392, 64.1388)
  line L102 (-72.6392, 64.1388) -> (-75.8302, 64.7464)
  line L103 (-75.8302, 64.7464) -> (-79.0233, 65.3246)
  line L104 (-79.0233, 65.3246) -> (-82.2185, 65.8733)
  line L105 (-82.2185, 65.8733) -> (-85.4157, 66.3926)
  line L106 (-85.4157, 66.3926) -> (-88.615, 66.8825)
  line L107 (-88.615, 66.8825) -> (-91.8156, 67.3528)
  line L108 (-91.8156, 67.3528) -> (-95.019, 67.7838)
  line L109 (-95.019, 67.7838) -> (-98.2251, 68.1756)
  line L110 (-53.5307, 59.9535) -> (-42.0166, 48.4395)
  line L111 (-53.5307, 59.9535) -> (-37.2474, 59.9535) construction
  point P0 (-8.426, 47.3224)
  dimension "d96" = 40
  dimension "d97" = 45
  constraint vertical L0
  constraint coincident L95 L0.start
  constraint coincident L73 L0.end
  constraint horizontal L111
  constraint coincident L95.end L96.start
  constraint coincident L73 L110.end
  measures "d96" distance of L0 P0
  measures "d97" angle of L110 L111
extrude "Extrude2''''" cut sketch "Sketch8" along normal blind 230 contours L0 L73 L110 bodies 2 in component "Component"
sketch "Sketch9" plane through (0, -145, 0) normal (0, -1, 0) x (1, 0, 0)
  line L0 (85.1135, -2.8201) -> (85.1135, -9.0163)
  line L1 (85.1135, -9.0163) -> (91.5229, -9.2295)
  line L2 (91.5229, -9.2295) -> (85.1135, -2.8201)
  line L3 (35.3144, 10.5067) -> (32.1062, 10.869)
  line L4 (32.1062, 10.869) -> (28.8953, 11.1921)
  line L5 (28.8953, 11.1921) -> (25.6816, 11.476)
  line L6 (25.6816, 11.476) -> (22.4652, 11.7206)
  line L7 (22.4652, 11.7206) -> (19.246, 11.926)
  line L8 (19.246, 11.926) -> (16.0241, 12.0922)
  line L9 (16.0241, 12.0922) -> (12.8008, 12.2387)
  line L10 (12.8008, 12.2387) -> (9.5755, 12.3558)
  line L11 (9.5755, 12.3558) -> (6.3474, 12.4336)
  line L12 (6.3474, 12.4336) -> (3.1152, 12.4526)
  line L13 (3.1152, 12.4526) -> (-0.1211, 12.4128)
  line L14 (-0.1211, 12.4128) -> (-3.3643, 12.2748)
  line L15 (-3.3643, 12.2748) -> (-6.6136, 12.0485)
  line L16 (-6.6136, 12.0485) -> (-9.8712, 11.7045)
  line L17 (-9.8712, 11.7045) -> (-13.1356, 11.2624)
  line L18 (-13.1356, 11.2624) -> (-16.4076, 10.7124)
  line L19 (-16.4076, 10.7124) -> (-19.6885, 10.0349)
  line L20 (-19.6885, 10.0349) -> (-22.9804, 9.2004)
  line L21 (-22.9804, 9.2004) -> (-26.284, 8.1991)
  line L22 (-26.284, 8.1991) -> (-27.9436, 7.5856)
  line L23 (-27.9436, 7.5856) -> (-29.6101, 6.8741)
  line L24 (-29.6101, 6.8741) -> (-31.2876, 6.0056)
  line L25 (-31.2876, 6.0056) -> (-32.983, 4.882)
  line L26 (-32.983, 4.882) -> (-34.3525, 3.7651)
  line L27 (-34.3525, 3.7651) -> (-35.0466, 3.1433)
  line L28 (-35.0466, 3.1433) -> (-35.7385, 2.4129)
  line L29 (-35.7385, 2.4129) -> (-36.0972, 1.9352)
  line L30 (-36.0972, 1.9352) -> (-36.2873, 1.6133)
  line L31 (-36.2873, 1.6133) -> (-36.3816, 1.3932)
  line L32 (-36.3816, 1.3932) -> (-36.4861, 1.0259)
  line L33 (-36.4861, 1.0259) -> (-36.4605, 0.265)
  line L34 (-36.4605, 0.265) -> (-36.3957, 0.0633)
  line L35 (-36.3957, 0.0633) -> (-36.2502, -0.2525)
  line L36 (-36.2502, -0.2525) -> (-35.9566, -0.7068)
  line L37 (-35.9566, -0.7068) -> (-35.3615, -1.3596)
  line L38 (-35.3615, -1.3596) -> (-34.7442, -1.8366)
  line L39 (-34.7442, -1.8366) -> (-33.4961, -2.4562)
  line L40 (-33.4961, -2.4562) -> (-31.914, -2.9513)
  line L41 (-31.914, -2.9513) -> (-30.3263, -3.3679)
  line L42 (-30.3263, -3.3679) -> (-28.7346, -3.7257)
  line L43 (-28.7346, -3.7257) -> (-27.138, -4.0148)
  line L44 (-27.138, -4.0148) -> (-23.9353, -4.4556)
  line L45 (-23.9353, -4.4556) -> (-20.7278, -4.8278)
  line L46 (-20.7278, -4.8278) -> (-17.5162, -5.1411)
  line L47 (-17.5162, -5.1411) -> (-14.3018, -5.4151)
  line L48 (-14.3018, -5.4151) -> (-11.0841, -5.6401)
  line L49 (-11.0841, -5.6401) -> (-7.8642, -5.8357)
  line L50 (-7.8642, -5.8357) -> (-4.6423, -6.0019)
  line L51 (-4.6423, -6.0019) -> (-1.4183, -6.1386)
  line L52 (-1.4183, -6.1386) -> (1.8063, -6.2655)
  line L53 (1.8063, -6.2655) -> (8.2584, -6.4801)
  line L54 (8.2584, -6.4801) -> (11.4851, -6.5775)
  line L55 (11.4851, -6.5775) -> (17.9371, -6.7921)
  line L56 (17.9371, -6.7921) -> (21.1632, -6.8994)
  line L57 (21.1632, -6.8994) -> (24.3892, -7.0067)
  line L58 (24.3892, -7.0067) -> (27.6152, -7.114)
  line L59 (27.6152, -7.114) -> (30.8412, -7.2213)
  line L60 (30.8412, -7.2213) -> (34.0673, -7.3285)
  line L61 (34.0673, -7.3285) -> (37.2933, -7.4358)
  line L62 (37.2933, -7.4358) -> (40.5193, -7.5431)
  line L63 (40.5193, -7.5431) -> (43.7453, -7.6504)
  line L64 (43.7453, -7.6504) -> (46.9713, -7.7577)
  line L65 (46.9713, -7.7577) -> (50.1974, -7.865)
  line L66 (50.1974, -7.865) -> (53.4234, -7.9723)
  line L67 (53.4234, -7.9723) -> (56.6494, -8.0795)
  line L68 (56.6494, -8.0795) -> (59.8754, -8.1868)
  line L69 (59.8754, -8.1868) -> (63.1015, -8.2941)
  line L70 (63.1015, -8.2941) -> (66.3275, -8.4014)
  line L71 (66.3275, -8.4014) -> (69.5535, -8.5087)
  line L72 (69.5535, -8.5087) -> (72.7795, -8.616)
  line L73 (72.7795, -8.616) -> (76.0056, -8.7233)
  line L74 (76.0056, -8.7233) -> (79.2323, -8.8207)
  line L75 (79.2323, -8.8207) -> (98.5884, -9.4645)
  line L76 (98.5884, -9.4645) -> (101.8144, -9.5717)
  line L77 (101.8144, -9.5717) -> (105.0405, -9.679)
  line L78 (105.0405, -9.679) -> (111.4925, -9.8936)
  line L79 (111.4925, -9.8936) -> (114.7185, -10.0009)
  line L80 (114.7185, -10.0009) -> (122.7836, -10.2691)
  line L81 (122.7836, -10.2691) -> (125.1135, -10.3466)
  line L82 (125.1135, -10.3466) -> (122.8282, -9.6314)
  line L83 (122.8282, -9.6314) -> (121.2454, -9.1461)
  line L84 (121.2454, -9.1461) -> (119.6632, -8.651)
  line L85 (119.6632, -8.651) -> (118.0804, -8.1657)
  line L86 (118.0804, -8.1657) -> (114.9147, -7.1951)
  line L87 (114.9147, -7.1951) -> (111.747, -6.254)
  line L88 (111.747, -6.254) -> (108.5786, -5.3226)
  line L89 (108.5786, -5.3226) -> (105.4096, -4.4011)
  line L90 (105.4096, -4.4011) -> (102.2384, -3.5089)
  line L91 (102.2384, -3.5089) -> (99.0666, -2.6266)
  line L92 (99.0666, -2.6266) -> (95.8934, -1.764)
  line L93 (95.8934, -1.764) -> (92.7195, -0.9111)
  line L94 (92.7195, -0.9111) -> (89.5435, -0.0876)
  line L95 (89.5435, -0.0876) -> (86.3669, 0.726)
  line L96 (86.3669, 0.726) -> (83.1882, 1.5102)
  line L97 (83.1882, 1.5102) -> (80.0088, 2.2846)
  line L98 (80.0088, 2.2846) -> (76.8274, 3.0295)
  line L99 (76.8274, 3.0295) -> (73.6453, 3.7647)
  line L100 (73.6453, 3.7647) -> (70.4618, 4.4802)
  line L101 (70.4618, 4.4802) -> (67.2762, 5.1663)
  line L102 (67.2762, 5.1663) -> (64.0893, 5.8328)
  line L103 (64.0893, 5.8328) -> (60.9003, 6.4698)
  line L104 (60.9003, 6.4698) -> (57.7093, 7.0774)
  line L105 (57.7093, 7.0774) -> (54.5162, 7.6556)
  line L106 (54.5162, 7.6556) -> (51.321, 8.2044)
  line L107 (51.321, 8.2044) -> (48.1238, 8.7237)
  line L108 (48.1238, 8.7237) -> (44.9246, 9.2136)
  line L109 (44.9246, 9.2136) -> (41.7239, 9.6838)
  line L110 (41.7239, 9.6838) -> (38.5205, 10.1149)
  line L111 (38.5205, 10.1149) -> (35.3144, 10.5067)
  line L112 (85.1135, -9.0163) -> (85.1135, 1.0412)
  constraint vertical L112
  constraint coincident L0.end L1.start
  constraint coincident L97 L112.end
extrude "Extrude3'''" cut sketch "Sketch9" along normal blind 4 contours L0 L1 L2 L75 L112 | L2 L75 L76 L77 L78 L79 L80 L81 L82 L83 L84 L85 L86 L87 L88 L89 L90 L91 L92 L93 L94 L95 L96 L112 bodies 2 in component "Component"
sketch "Sketch10" plane through (0, -375, 0) normal (0, 1, 0) x (-1, 0, 0)
  line L0 (-85.1135, -9.0163) -> (-85.1135, -2.8201)
  line L1 (-85.1135, -2.8201) -> (-91.5229, -9.2295)
  line L2 (-91.5229, -9.2295) -> (-85.1135, -9.0163)
  line L3 (-85.1135, 1.0352) -> (-85.1135, -9.0163)
  line L4 (-85.1135, -9.0163) -> (-98.5884, -9.4645)
  line L5 (-98.5884, -9.4645) -> (-101.8144, -9.5717)
  line L6 (-101.8144, -9.5717) -> (-105.0405, -9.679)
  line L7 (-105.0405, -9.679) -> (-111.4925, -9.8936)
  line L8 (-111.4925, -9.8936) -> (-114.7185, -10.0009)
  line L9 (-114.7185, -10.0009) -> (-122.7836, -10.2691)
  line L10 (-122.7836, -10.2691) -> (-125.1135, -10.3466)
  line L11 (-125.1135, -10.3466) -> (-122.8282, -9.6314)
  line L12 (-122.8282, -9.6314) -> (-121.2454, -9.1461)
  line L13 (-121.2454, -9.1461) -> (-119.6632, -8.651)
  line L14 (-119.6632, -8.651) -> (-118.0804, -8.1657)
  line L15 (-118.0804, -8.1657) -> (-114.9147, -7.1951)
  line L16 (-114.9147, -7.1951) -> (-111.747, -6.254)
  line L17 (-111.747, -6.254) -> (-108.5786, -5.3226)
  line L18 (-108.5786, -5.3226) -> (-105.4096, -4.4011)
  line L19 (-105.4096, -4.4011) -> (-102.2384, -3.5089)
  line L20 (-102.2384, -3.5089) -> (-99.0666, -2.6266)
  line L21 (-99.0666, -2.6266) -> (-95.8934, -1.764)
  line L22 (-95.8934, -1.764) -> (-92.7195, -0.9111)
  line L23 (-92.7195, -0.9111) -> (-89.5435, -0.0876)
  line L24 (-89.5435, -0.0876) -> (-86.3669, 0.726)
  line L25 (-86.3669, 0.726) -> (-85.1135, 1.0352)
extrude "Extrude4'" cut sketch "Sketch10" along normal blind 4 bodies 2 in component "Component"
mirror "Mirror1" about plane through (0, 0, 0) normal (0, 1, 0) of "Extrude2''''", "Extrude3'''", "Extrude4'" in component "Component"
ref_plane "WorkPlane3" through (-26.4605, 0, -70.9227) normal (-1, 0, 0) x (0, 0, -1)
sketch "Sketch12" plane through (-26.4605, 0, -70.9227) normal (-1, 0, 0) x (0, 1, 0)
  line L0 (45, -2.925) -> (45, 43.8327)
  line L1 (35, 43.4816) -> (106.1111, 114.5927)
  line L2 (106.1111, 114.5927) -> (106.1111, 129.5927)
  line L3 (33.5858, 44.8958) -> (104.1111, 115.4211)
  line L4 (104.1111, 115.4211) -> (104.1111, 129.5927)
  line L5 (106.1111, 129.5927) -> (104.1111, 129.5927)
  line L6 (-97, 115.8327) -> (-97, 130.8327)
  line L7 (-95, 116.6612) -> (-95, 130.8327)
  line L8 (-97, 130.8327) -> (-95, 130.8327)
  line L9 (-33.4462, 45.0392) -> (-95, 116.6612)
  line L10 (-35, 43.4816) -> (-97, 115.8327)
  line L11 (35, 43.4816) -> (-35, 43.4816)
  line L12 (-35, 43.4816) -> (-35, 45.6308)
  line L13 (-35, 45.6308) -> (35, 45.6308)
  line L14 (35, 45.6308) -> (35, 43.4816)
  dimension "d113" = 15
  dimension "d115" = -2
  dimension "d151" = 70
  dimension "d152" = 10
  constraint vertical L2
  constraint horizontal L11
  constraint vertical L12
  constraint horizontal L13
  constraint vertical L14
  measures "d113" distance of L1.end L2.end
  measures "d151" distance of L1.start L10.start
  measures "d152" distance of L0 L14
extrude "Extrude2'''''" add sketch "Sketch12" against normal blind 30 separate body makes body 7
sketch "Sketch13" plane through (0, -97, 0) normal (0, -1, 0) x (1, 0, 0)
  line L0 (-26.4605, -186.7554) -> (-26.4605, -201.7554)
  line L1 (-26.4605, -201.7554) -> (3.5395, -201.7554)
  line L2 (3.5395, -201.7554) -> (3.5395, -186.7554)
  line L3 (3.5395, -186.7554) -> (-26.4605, -186.7554)
  circle A0 centre (-11.4605, -194.2554) radius 1.5
  dimension "d118" = 3
  dimension "d134" = 15
  dimension "d135" = 7.5
  measures "d118" diameter of A0
  measures "d134" distance of L2 A0.centre
  measures "d135" distance of L1 A0.centre
extrude "Extrude3''''" cut sketch "Sketch13" against normal up to surface (203.1111 mm away) contours A0 bodies 7
copy_body "Body->Comp3" bodies 7 removing the originals makes body 8 in component "Component'''''"
ref_plane "WorkPlane4" through (-11.4605, -97, -194.2554) normal (0, -1, 0) x (0, 0, -1)
sketch "Sketch14" plane through (-1.4605, -97, -204.2554) normal (0, -1, 0) x (1, 0, 0)
  circle A0 centre (-10, 10) radius 30
  line L0 (-25, 17.5) -> (-25, 2.5)
  line L1 (-25, 2.5) -> (5, 2.5)
  dimension "d122" = 60
  dimension "d136" = 15
  dimension "d137" = 7.5
  measures "d122" diameter of A0
  measures "d136" distance of A0.centre L0
  measures "d137" distance of A0.centre L1
extrude "Extrude4''" add sketch "Sketch14" along normal blind 20 separate body makes body 9
copy_body "Body->Comp4" bodies 9 removing the originals makes body 10 in component "Component''''''"
move_body "Move1" bodies 10 to x (1, 0, 0) y (0, 1, 0) z (0, 0, 1) at (0, -1, 0) in component "Component''''''"
sketch "Sketch15" plane through (0, 0, 0) normal (0, 1, 0) x (1, 0, 0)
  line L0 (354.4293, 66.7768) -> (377.8488, 142.5104)
  line L1 (373.5366, 60.8681) -> (396.9561, 136.6018)
  line L2 (354.4293, 66.7768) -> (373.5366, 60.8681)
  line L3 (377.8488, 142.5104) -> (396.9561, 136.6018)
  circle A0 centre (384.4482, 130.0025) radius 1.5
  dimension "d125" = 20
  dimension "d126" = 10
  dimension "d127" = 10
  dimension "d130" = 3
  measures "d126" distance of L0 A0.centre
  measures "d127" distance of L3 A0.centre
  measures "d130" diameter of A0